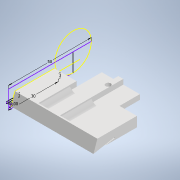
# Autodesk Inventor part: podsta
Saved by Autodesk Inventor 2022 (Build 260153000, 153)
## iProperties
Created: 2022-12-13
Part Number: podsta
Material: Generic
Document SubType Name: Modeling
Designer: komputer
Density: 1 g/cm^3
Appearance: Default
Author: komputer
Autodesk Inventor part; units mm, degrees
ref_plane "YZ Plane" through (0, 0, 0) normal (1, 0, 0) x (0, 1, 0)
ref_plane "XZ Plane" through (0, 0, 0) normal (0, 1, 0) x (-1, 0, 0)
ref_plane "XY Plane" through (0, 0, 0) normal (0, 0, 1) x (1, 0, 0)
sketch "Sketch1" plane through (0, 0, 0) normal (0, 1, 0) x (-1, 0, 0)
  line L0 (-25, -25) -> (25, -25)
  line L1 (25, -25) -> (25, 25)
  line L2 (25, 25) -> (-25, 25)
  line L3 (-25, 25) -> (-25, -25)
  point P0 (0, 0)
  dimension "d2" = 50
  dimension "d3" = 50
  constraints: 8 end point, 2 parallel, 1 horizontal, 1 perpendicular
  measures "d2" distance of L2.end L1.end
  measures "d3" distance of L1.end L0.end
extrude "Extrusion1" add sketch "Sketch1" along normal blind 4
sketch "Sketch2" plane through (0, 4, 0) normal (0, 1, 0) x (1, 0, 0)
  line L0 (-25, 25) -> (-25, -25) projected
  line L1 (-25, -25) -> (25, -25) projected
  line L2 (25, -25) -> (25, 25) projected
  line L3 (25, 25) -> (-25, 25) projected
  line L4 (-25, -25) -> (25, -25) projected
  line L5 (0, -25) -> (0, 25)
  line L6 (25, 25) -> (-25, 25) projected
  line L7 (0, -25) -> (-1.5, -25)
  line L8 (-1.5, -25) -> (1.5, -25)
  line L9 (1.5, -25) -> (1.5, 25)
  line L10 (1.5, 25) -> (-1.5, 25)
  line L11 (-1.5, 25) -> (-1.5, -25)
  line L12 (1.5, 9.2284) -> (-1.5, 9.2284)
  line L13 (1.5, 9.2284) -> (-1.5, 9.2284)
  line L14 (-1.5, 9.2284) -> (-1.5, 25)
  line L15 (-1.5, 25) -> (1.5, 25)
  line L16 (1.5, 25) -> (1.5, 9.2284)
  point P0 (0, 0)
  point P1 (1.5, 25)
  dimension "d6" = 1.5
  dimension "d7" = 3
  constraints: 22 end point, 4 parallel, 4 point on line, 3 perpendicular, 2 horizontal, 2 midpoint
  measures "d6" distance of L5.start L7.end
  measures "d7" distance of L10.end L9.end
extrude "Extrusion2" add sketch "Sketch2" along normal blind 3 contours L3 L5 L12 L11 | L3 L9 L12 L5
sketch "Sketch3" plane through (0, 4, 0) normal (0, 1, 0) x (1, 0, 0)
  line L0 (1.5, 25) -> (1.5, 9.2284) projected
  line L1 (1.5, 9.2284) -> (-1.5, 9.2284) projected
  line L2 (-1.5, 9.2284) -> (-1.5, 25) projected
  line L3 (-1.5, 25) -> (-25, 25) projected
  line L4 (-25, 25) -> (-25, -25) projected
  line L5 (-25, -25) -> (25, -25) projected
  line L6 (25, -25) -> (25, 25) projected
  line L7 (25, 25) -> (1.5, 25) projected
  line L8 (11.5, 24.5) -> (11.5, 9.7) projected
  line L9 (-11.5, 9.7) -> (-11.5, 24.5) projected
  line L10 (25, 25) -> (1.5, 25) projected
  line L11 (25, 25) -> (11.5, 25)
  line L12 (11.5, 25) -> (11.5, 9.7)
  line L13 (11.5, 9.7) -> (25, 9.7)
  line L14 (25, 9.7) -> (25, 25)
  line L15 (-11.5, 9.7) -> (-25, 9.7)
  line L16 (-25, 9.7) -> (-25, 25)
  line L17 (-25, 25) -> (-11.5, 25)
  line L18 (-11.5, 25) -> (-11.5, 9.7)
  point P0 (0, 0)
  constraints: 16 end point, 4 parallel, 2 horizontal, 2 perpendicular
extrude "Extrusion3" cut sketch "Sketch3" against normal blind 10 contours L7 L6 L13 L8 L12 | L18 L9 L15 L4 L3
sketch "Sketch4" plane through (0, 0, 0) normal (0, -1, 0) x (1, 0, 0)
  line L0 (-11.5, -9.7) -> (-11.5, -25) projected
  line L1 (11.5, -25) -> (-11.5, -25) projected
  line L2 (11.5, -25) -> (11.5, -9.7) projected
  line L3 (11.5, -9.7) -> (25, -9.7) projected
  line L4 (25, 25) -> (25, -9.7) projected
  line L5 (-25, 25) -> (25, 25) projected
  line L6 (-25, -9.7) -> (-25, 25) projected
  line L7 (-25, -9.7) -> (-11.5, -9.7) projected
  point P0 (0, 0)
extrude "Extrusion4" cut sketch "Sketch4" against normal blind 1
sketch "Sketch5" plane through (-25, 4, 25) normal (0, 0, 1) x (1, 0, 0)
  line L0 (0, -3) -> (50, -3) projected
  line L1 (50, -3) -> (50, 0) projected
  line L2 (0, 0) -> (50, 0) projected
  line L3 (0, -3) -> (0, 0) projected
  line L4 (0, 0) -> (50, 0) projected
  line L5 (0, 0) -> (50, 0)
  line L6 (50, 0) -> (50, 3)
  line L7 (50, 3) -> (0, 3)
  line L8 (0, 3) -> (0, 0)
  point P0 (25, -4)
  dimension "d14" = 3
  constraints: 8 end point, 2 parallel, 1 horizontal, 1 perpendicular
  measures "d14" distance of L6.end L5.end
extrude "Extrusion5" add sketch "Sketch5" against normal up to surface (34.7 mm away) contours L8 L7 L6 L2
sketch "Sketch6" plane through (11.5, 4, -9.7) normal (0, 0, -1) x (-1, 0, 0)
  line L0 (-13.5, -3) -> (0, -3) projected
  line L1 (0, 0) -> (0, -3) projected
  line L2 (10, 0) -> (0, 0) projected
  line L3 (10, 3) -> (10, 0) projected
  line L4 (10, 3) -> (-13.5, 3) projected
  line L5 (-13.5, -3) -> (-13.5, 3) projected
  line L6 (23, -3) -> (36.5, -3) projected
  line L7 (36.5, 3) -> (36.5, -3) projected
  line L8 (36.5, 3) -> (13, 3) projected
  line L9 (13, 0) -> (13, 3) projected
  line L10 (23, 0) -> (13, 0) projected
  line L11 (23, 0) -> (23, -3) projected
  line L12 (0, 0.5) -> (0, 11.5) projected
  line L13 (23, 11.5) -> (23, 0.5) projected
  line L14 (10, 0) -> (0, 0) projected
  line L15 (0, 11.5) -> (0, 0)
  line L16 (23, 11.5) -> (23, 0)
  line L17 (0, 0) -> (0, -3) projected
  line L18 (10, 3) -> (-13.5, 3) projected
  line L19 (0, 0) -> (10, 0)
  line L20 (10, 0) -> (10, 3)
  line L21 (10, 3) -> (0, 3)
  line L22 (0, 3) -> (0, 0)
  line L23 (13, 0) -> (13, 3) projected
  line L24 (23, 0) -> (23, -3) projected
  line L25 (13, 3) -> (23, 3)
  line L26 (23, 3) -> (23, 0)
  line L27 (23, 0) -> (13, 0)
  line L28 (13, 0) -> (13, 3)
  point P0 (11.5, -4)
  point P1 (23, 0.5)
  point P2 (0, 3)
  constraints: 20 end point, 4 parallel, 3 perpendicular, 2 horizontal, 1 vertical
extrude "Extrusion6" cut sketch "Sketch6" against normal blind 20 contours L15 L12 L4 L3 L2 | L10 L9 L8 L13 L16
sketch "Sketch7" plane through (11.5, 4, 10.3) normal (0, 0, -1) x (-1, 0, 0)
  arc A0 (0, 2.75) -> (10, 2.7503) centre (4.9999, 5.9206) ccw projected
  arc A1 (13, 2.75) -> (23, 2.7497) centre (18.0001, 5.9203) ccw projected
  line L0 (0, 0) -> (10, 0) projected
  line L1 (5, 0) -> (5, -0.3289)
  line L2 (5, -0.3289) -> (19.1354, -0.3289)
  circle A2 centre (4.9999, 5.9206) radius 6.2495
  circle A3 centre (18.0001, 5.9203) radius 6.2492
  line L3 (0, 3) -> (-13.5, 3) projected
  line L4 (0, 3) -> (10, 3)
  line L5 (10, 3) -> (10, 0)
  line L6 (10, 0) -> (0, 0)
  line L7 (0, 0) -> (0, 3)
  line L8 (13, 0) -> (13, 3) projected
  line L9 (23, 3) -> (23, 0) projected
  line L10 (13, 0) -> (23, 0)
  line L11 (23, 0) -> (23, 3)
  line L12 (23, 3) -> (13, 3)
  line L13 (13, 3) -> (13, 0)
  point P0 (11.5, -4)
  point P1 (20.0008, 0)
  point P2 (23, 2.1715)
  point P3 (15.9994, 0)
  point P4 (13, 2.1717)
  point P5 (10, 2.1715)
  point P6 (7.0007, 0)
  point P7 (0, 2.1713)
  point P8 (2.9992, 0)
  constraints: 20 end point, 4 parallel, 3 perpendicular, 2 coincident, 2 horizontal, 1 centre point, 1 midpoint, 1 tangent, 1 vertical, 3 other
extrude "Extrusion7" add sketch "Sketch7" along normal blind 16 contours A2 L0 L7 | A2 L5 L0 | A3 L10 L8 | A3 L9 L10
chamfer "Chamfer1" distance 3 angle 45 2 edges at (6.5, 7, 10.3) (-6.5, 7, 10.3)
sketch "Sketch8" plane through (-25, 7, -9.7) normal (-1, 0, 0) x (0, 0, 1)
  circle A0 centre (-11.34, 3) radius 8 projected
  line L0 (0, -6) -> (34.7, -6) projected
  line L1 (34.7, -6) -> (34.7, 0) projected
  line L2 (34.7, 0) -> (0, 0) projected
  line L3 (0, 0) -> (0, -6) projected
  line L4 (-11.34, 3) -> (-19.34, 3)
  line L5 (-19.34, 3) -> (-22.34, 3)
  line L6 (-22.34, 3) -> (27.66, 3)
  line L7 (0, -6) -> (34.7, -6) projected
  line L8 (34.7, -6) -> (27.66, -6)
  line L9 (27.66, -6) -> (27.66, 9.5427)
  line L10 (27.66, 9.5427) -> (34.7, 9.5427)
  line L11 (34.7, 9.5427) -> (34.7, -6)
  point P0 (9.7, -7)
  point P1 (27.66, 0)
  dimension "d24" = 3
  dimension "d25" = 50
  constraints: 14 end point, 2 parallel, 2 point on line, 1 horizontal, 1 horizontal alignment, 1 perpendicular, 1 other
  measures "d24" distance of L4.end L5.end
  measures "d25" distance of L5.end L6.end
extrude "Extrusion8" cut sketch "Sketch8" against normal through all contours L9 L2 L1 L0
sketch "Sketch9" plane through (25, 1, -9.7) normal (1, 0, 0) x (0, 0, -1)
  line L0 (-27.66, 6) -> (-27.66, 0) projected
  line L1 (-27.66, 0) -> (0, 0) projected
  line L2 (0, 0) -> (0, 6) projected
  line L3 (-27.66, 6) -> (0, 6) projected
  line L4 (-27.66, 0.31) -> (-25.7682, 0.01) projected
  line L5 (-25.7682, 0.01) -> (-14.0234, 0.01) projected
  line L6 (-14.0234, 0.01) -> (-14.0234, 0.61) projected
  line L7 (-25.7682, 0.61) -> (-14.0234, 0.61) projected
  line L8 (-25.7682, 0.61) -> (-27.66, 0.31) projected
  line L9 (-27.66, 0) -> (-27.66, 6) projected
  line L10 (-14.0234, 0.61) -> (-27.66, 0.61)
  line L11 (-27.66, 0.61) -> (-27.66, 1.22)
  line L12 (-27.66, 1.22) -> (-14.0234, 1.22)
  line L13 (-14.0234, 1.22) -> (-14.0234, 0.61)
  point P0 (-9.7, -1)
  point P1 (-27.66, 1.22)
  dimension "d28" = 0.61
  constraints: 8 end point, 2 parallel, 1 horizontal, 1 perpendicular, 1 point on line, 1 other
  measures "d28" distance of L10.end L11.end
extrude "Extrusion9" cut sketch "Sketch9" against normal through all contours L12 L13 L7 L10 L0
sketch "Sketch10" plane through (25, 1, -9.7) normal (1, 0, 0) x (0, 0, -1)
  line L0 (-27.66, 0.31) -> (-25.7682, 0.01) projected
  line L1 (-25.7682, 0.01) -> (-14.0234, 0.01) projected
  line L2 (-14.0234, 0.01) -> (-14.0234, 0.61) projected
  line L3 (-25.7682, 0.61) -> (-14.0234, 0.61) projected
  line L4 (-25.7682, 0.61) -> (-27.66, 0.31) projected
  line L5 (-14.0234, 1.22) -> (-14.0234, 0.61) projected
  line L6 (-27.66, 0) -> (0, 0) projected
  line L7 (0, 0) -> (0, 6) projected
  line L8 (-27.66, 6) -> (0, 6) projected
  line L9 (-27.66, 6) -> (-27.66, 1.22) projected
  line L10 (-27.66, 1.22) -> (-14.0234, 1.22) projected
  line L11 (-25.7682, 0.61) -> (-25.7682, 6)
  line L12 (-27.66, 6) -> (0, 6) projected
  line L13 (-19.9, 5.7) -> (-19.9, 6.1)
  line L14 (15.3, 6) -> (-23, 6) projected
  line L15 (-19.9, 6) -> (-20.9, 6)
  line L16 (-20.9, 6) -> (-23.9, 6)
  line L17 (-25.7682, 0.61) -> (-23.9, 6)
  line L18 (-14.0234, 0.61) -> (-27.66, 0.61) projected
  line L19 (-27.66, 0.61) -> (-27.66, 0) projected
  point P0 (-9.7, -1)
  point P1 (-25.5568, 1.22)
  dimension "d31" = 1
  dimension "d32" = 3
  constraints: 10 end point, 5 point on line, 1 perpendicular, 1 vertical, 2 other
  measures "d31" distance of L15.start L15.end
  measures "d32" distance of L15.end L16.end
extrude "Extrusion10" cut sketch "Sketch10" against normal through all contours L11 L8 L17 L10 | L10 L9 L8 L11
sketch "Sketch11" plane through (0, 1, 0) normal (0, -1, 0) x (1, 0, 0)
  circle A0 centre (0, -17.35) radius 1.5 projected
  line L0 (3.695, -17.35) -> (1.8475, -14.15) projected
  line L1 (1.8475, -20.55) -> (3.695, -17.35) projected
  line L2 (-1.8475, -20.55) -> (1.8475, -20.55) projected
  line L3 (-3.695, -17.35) -> (-1.8475, -20.55) projected
  line L4 (-1.8475, -14.15) -> (-3.695, -17.35) projected
  line L5 (1.8475, -14.15) -> (-1.8475, -14.15) projected
  circle A1 centre (0, -17.35) radius 1.5 projected
  line L6 (-25, -10.04) -> (-25, -32.04) projected
  point P0 (0, 0)
extrude "Extrusion11" cut sketch "Sketch11" against normal through all contours A0
chamfer "Chamfer2" distance 1 angle 45 1 edges at (-1.5, 1, -17.35)
sketch "Sketch12" plane through (-25, 1, -9.7) normal (-1, 0, 0) x (0, 0, 1)
  line L0 (25.5568, 1.22) -> (23.9, 6) projected
  line L1 (23.9, 6) -> (0, 6) projected
  line L2 (0, 6) -> (0, 0) projected
  line L3 (0, 0) -> (27.66, 0) projected
  line L4 (27.66, 0) -> (27.66, 0.61) projected
  line L5 (27.66, 0.61) -> (14.0234, 0.61) projected
  line L6 (14.0234, 0.61) -> (14.0234, 1.22) projected
  line L7 (14.0234, 1.22) -> (25.5568, 1.22) projected
  circle A0 centre (-11.34, 9) radius 11 projected
  line L8 (-22.34, 9) -> (27.66, 9)
  line L9 (27.66, 9) -> (27.66, -12.93)
  line L10 (-11.34, 9) -> (-11.34, -2)
  line L11 (-11.34, -2) -> (27.66, -1.965)
  line L12 (14.0234, 1.22) -> (25.5568, 1.22) projected
  line L13 (27.66, -1.3745) -> (14.0234, 1.22)
  line L14 (14.0234, 1.22) -> (14.0795, 1.5147)
  line L15 (14.0234, 1.22) -> (13.9673, 0.9253)
  line L16 (14.0795, 1.5147) -> (28.9229, -1.3094)
  line L17 (13.9673, 0.9253) -> (29.035, -1.9638)
  line L18 (25.5568, 1.22) -> (24.566, 4.0785)
  line L19 (25.5568, 1.22) -> (23.9, 6) projected
  line L20 (25.5568, 1.22) -> (26.2577, -0.8023)
  point P0 (9.7, -1)
  point P1 (15.6117, 0.61)
  point P2 (14.0234, 0.9145)
  point P3 (15.6285, 1.22)
  dimension "d40" = 0.3
  dimension "d41" = 0.3
  constraints: 22 end point, 4 point on line, 2 perpendicular, 2 point on circle, 2 vertical, 1 horizontal, 1 midpoint, 1 parallel
  measures "d40" distance of L6.end L14.end
  measures "d41" distance of L6.end L15.end
extrude "Extrusion12" add sketch "Sketch12" against normal blind 50 contours L20 L5 L16 L7 | L20 L3 L16 L5 | L20 L16 L3 | L17 L5 L6
sketch "Sketch13" plane through (-25, 1, -9.7) normal (-1, 0, 0) x (0, 0, 1)
  line L0 (18.8347, 0.61) -> (15.6117, 0.61) projected
  line L1 (15.6117, 0.61) -> (14.0234, 0.9145) projected
  line L2 (14.0234, 0.9145) -> (14.0234, 1.22) projected
  line L3 (14.0234, 1.22) -> (15.6285, 1.22) projected
  line L4 (15.6285, 1.22) -> (18.8347, 0.61) projected
  line L5 (25.7682, 0.61) -> (23.9, 6) projected
  line L6 (23.9, 6) -> (0, 6) projected
  line L7 (0, 6) -> (0, 0) projected
  line L8 (0, 0) -> (22.0408, 0) projected
  line L9 (22.0408, 0) -> (26.2577, -0.8023) projected
  line L10 (26.2577, -0.8023) -> (25.9796, 0) projected
  line L11 (25.9796, 0) -> (27.66, 0) projected
  line L12 (27.66, 0) -> (27.66, 0.61) projected
  line L13 (27.66, 0.61) -> (25.7682, 0.61) projected
  line L14 (14.0234, 0.9145) -> (14.0234, 1.22) projected
  line L15 (14.0234, 0.9145) -> (26.7141, -1.5188)
  line L16 (14.0234, 1.22) -> (15.6285, 1.22) projected
  line L17 (15.6285, 1.22) -> (29.31, -1.383)
  line L18 (14.0234, 0.9145) -> (13.2268, 1.0673)
  line L19 (13.2268, 1.0673) -> (13.3704, 1.8159)
  line L20 (15.6285, 1.22) -> (13.3396, 1.6555)
  line L21 (25.9796, 0) -> (27.66, 0) projected
  line L22 (25.9796, 0) -> (25.7682, 0.61)
  line L23 (26.7141, -1.5188) -> (27.0047, -0.9444)
  point P0 (9.7, -1)
  point P1 (18.7931, 0)
  constraints: 14 end point, 3 point on line, 1 perpendicular
extrude "Extrusion13" cut sketch "Sketch13" against normal through all contours L17 L8 L15 L0 | L3 L2 L18 L19 L20 | L22 L13 L12 L11
sketch "Sketch14" plane through (-25, 1, -9.7) normal (-1, 0, 0) x (0, 0, 1)
  line L0 (26.2577, -0.8023) -> (23.9, 6) projected
  line L1 (23.9, 6) -> (0, 6) projected
  line L2 (0, 6) -> (0, 0) projected
  line L3 (0, 0) -> (18.7931, 0) projected
  line L4 (18.7931, 0) -> (13.2268, 1.0673) projected
  line L5 (13.2268, 1.0673) -> (13.3396, 1.6555) projected
  line L6 (13.3396, 1.6555) -> (26.2577, -0.8023) projected
  circle A0 centre (-11.34, 9) radius 11 projected
  line L7 (-22.34, 9) -> (27.66, 9)
  line L8 (-11.34, 9) -> (-11.34, -2)
  line L9 (-11.34, 9) -> (27.66, 9)
  line L10 (27.66, 9) -> (27.66, -2)
  line L11 (27.66, -2) -> (-11.34, -2)
  line L12 (-11.34, -2) -> (-11.34, 9)
  line L13 (4, 3) -> (-7.65, 3) projected
  line L14 (-7.65, 3) -> (-15.3, 3) projected
  line L15 (-15.3, 3) -> (0, 3) projected
  line L16 (0, 3) -> (4, 3) projected
  line L17 (4, 3) -> (20, 3) projected
  line L18 (20, 3) -> (4, 3) projected
  line L19 (0, 3) -> (-15.3, 3) projected
  line L20 (0, 3) -> (20, 3)
  line L21 (20, 3) -> (20, 2)
  line L22 (20, 2) -> (0, 2)
  line L23 (0, 2) -> (0, 3)
  line L24 (22.1715, 5.1715) -> (20, 3) projected
  line L25 (20, 3) -> (29.0462, 3)
  line L26 (29.0462, 3) -> (29.0462, 2)
  line L27 (29.0462, 2) -> (20, 2)
  line L28 (20, 2) -> (20, 3)
  line L29 (27.66, 2) -> (-2.34, 2)
  line L30 (-2.34, 2) -> (-2.34, -1)
  line L31 (-2.34, -1) -> (27.66, -1)
  line L32 (27.66, -1) -> (27.66, 2)
  line L33 (27.66, -1) -> (24.0847, 2)
  line L34 (26.2577, -0.8023) -> (23.9, 6) projected
  line L35 (24.0847, 2) -> (23.5108, 6)
  line L36 (23.9, 6) -> (0, 6) projected
  point P0 (9.7, -1)
  point P1 (24.0847, 2)
  point P2 (25.7792, 0.5781)
  dimension "d46" = 50
  dimension "d47" = 1
  dimension "d48" = 30
  dimension "d49" = 3
  dimension "d50" = 40
  constraints: 40 end point, 8 parallel, 5 horizontal, 5 point on line, 4 perpendicular, 2 point on circle, 1 vertical
  measures "d46" distance of L7.start L7.end
  measures "d47" distance of L20.end L21.end
  measures "d48" distance of L31.end L30.end
  measures "d49" distance of L30.end L29.end
  measures "d50" angle of L31 L33
extrude "Extrusion14" cut sketch "Sketch14" against normal through all contours L6 L5 L4 L3 L2 L22 L27 L33 L0 | L0 L33 L31 L30 L29 L2 L3 L4 L5 L6 | L33 L27 L0 | L27 L35 L25 L0 | L25 L35 L1 L0
body "Solid1"
